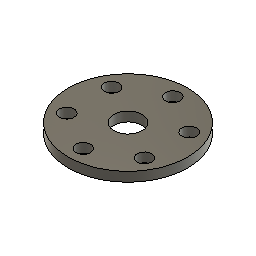
HubSpacer2 v3 (Autodesk Fusion 360 design; units mm, degrees)
Autodesk Fusion 360 part; units mm, degrees
sketch "Sketch1" plane through (0, 0, 0) normal (0, 1, 0) x (1, 0, 0)
  circle A0 centre (0, 0) radius 12.7
  circle A1 centre (0, 0) radius 9.525 construction
  circle A2 centre (-0.0005, 9.525) radius 1.55
  circle A3 centre (-8.2491, 4.7621) radius 1.55
  circle A4 centre (-8.2487, -4.7629) radius 1.55
  circle A5 centre (0.0005, -9.525) radius 1.55
  circle A6 centre (8.2491, -4.7621) radius 1.55
  circle A7 centre (8.2487, 4.7629) radius 1.55
  circle A8 centre (0, 0) radius 3
  dimension "d1" = 25.4
  dimension "d2" = 19.05
  dimension "d3" = 3.1
  dimension "d5" = 360
  dimension "d6" = 6
  constraint coincident A0.centre A1.centre
  constraint concentric A0 A1
  constraint coincident A1 A2.centre
  measures "d1" diameter of A0
  measures "d2" diameter of A1
  measures "d3" diameter of A2
  measures "d6" diameter of A8
extrude "Extrude1" add sketch "Sketch1" along normal blind 2
